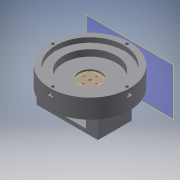
# Autodesk Inventor part: rotacion1_bottom
Saved by Autodesk Inventor 2018 (Build 220112000, 112)
## iProperties
Created: 2016-09-29
Part Number: rotacion1_bottom
Material: Generic
Document SubType Name: Modeling
Designer: Bardo91
Density: 1 g/cm^3
Appearance: Default
Author: Bardo91
Autodesk Inventor part; units mm, degrees
ref_plane "YZ Plane" through (0, 0, 0) normal (1, 0, 0) x (0, 1, 0)
ref_plane "XZ Plane" through (0, 0, 0) normal (0, 1, 0) x (-1, 0, 0)
ref_plane "XY Plane" through (0, 0, 0) normal (0, 0, 1) x (1, 0, 0)
sketch "Sketch1" plane through (0, 0, 0) normal (0, 0, 1) x (1, 0, 0)
  circle A0 centre (0, 0) radius 43
  circle A1 centre (0, 0) radius 50
  dimension "d0" = 86
  dimension "d1" = 100
  constraints: 2 centre point, 2 coincident
  measures "d0" diameter of A0
  measures "d1" diameter of A1
extrude "Extrusion1" add sketch "Sketch1" along normal blind 14
sketch "Sketch2" plane through (0, 0, 0) normal (0, 0, -1) x (-1, 0, 0)
  circle A0 centre (0, 0) radius 50.0172
  constraints: 1 centre point, 1 coincident
extrude "Extrusion2" add sketch "Sketch2" along normal blind 10
sketch "Sketch3" plane through (0, 0, -10) normal (0, 0, -1) x (-1, 0, 0)
  line L0 (0, 0) -> (0, 20)
  line L1 (0, 20) -> (-10, 20)
  line L2 (-10, 20) -> (-10, -20)
  line L3 (-10, -20) -> (31, -20)
  line L4 (31, -20) -> (31, 20)
  line L5 (31, 20) -> (0, 20)
  line L6 (-10, 20) -> (-10, 12.5)
  line L7 (-10, 12.5) -> (-17.5, 12.5)
  line L8 (-10, 12.5) -> (-10, 17.5)
  line L9 (-17.5, 17.5) -> (-17.5, 12.5)
  line L10 (-17.5, 12.5) -> (-17.5, -22.5)
  line L11 (-17.5, -22.5) -> (-32.5, -22.5)
  line L12 (-32.5, -22.5) -> (-32.5, 20)
  line L13 (-32.5, 20) -> (-17.5, 20)
  line L14 (31, -20) -> (31, -22.5)
  line L15 (31, -22.5) -> (38.5, -22.5)
  line L16 (38.5, -22.5) -> (38.5, 12.5)
  line L17 (38.5, 20) -> (31, 20)
  line L18 (-17.5, 20) -> (-10, 20)
  arc A0 (44.6514, -22.5) -> (45.8258, 20) centre (0, 0) ccw
  line L19 (38.5, -22.5) -> (44.6514, -22.5)
  line L20 (38.5, 20) -> (45.8258, 20)
  line L21 (31, 12.5) -> (38.5, 12.5)
  dimension "d6" = 20
  dimension "d7" = 10
  dimension "d8" = 40
  dimension "d9" = 41
  dimension "d10" = 7.5
  dimension "d11" = 7.5
  dimension "d13" = 35
  dimension "d14" = 15
  dimension "d16" = 7.5
  dimension "d24" = 2.5
  constraints: 44 end point, 10 perpendicular, 6 point on line, 5 vertical, 2 horizontal, 2 point on circle, 1 centre point, 1 coincident, 1 collinear
  measures "d6" distance of L0.start L0.end
  measures "d7" distance of L0.end L1.end
  measures "d8" distance of L1.end L2.end
  measures "d9" distance of L2.end L3.end
  measures "d10" distance of L1.end L6.end
  measures "d11" distance of L6.end L7.end
  measures "d13" distance of L7.end L10.end
  measures "d14" distance of L10.end L11.end
  measures "d16" distance of L14.end L15.end
  measures "d24" distance of L3.end L14.end
extrude "Extrusion3" add sketch "Sketch3" along normal blind 5 contours L5 L4 L3 L2 L1
extrude "Extrusion4" add sketch "Sketch3" along normal blind 25 contours L2 L7 L10 L11 L12 L13 L18 | L17 L20 A0 L19 L16 L21 L4
sketch "Sketch4" plane through (0, 0, -35) normal (0, 0, -1) x (-1, 0, 0)
  arc A0 (44.6514, -22.5) -> (45.8258, 20) centre (0, 0) ccw
  line L0 (45.8258, 20) -> (-32.5, 20)
  line L1 (-32.5, 20) -> (45.8258, 20) projected
  line L2 (-32.5, 20) -> (-32.5, -22.5)
  line L3 (-17.5, -22.5) -> (-32.5, -22.5) projected
  line L4 (-32.5, -22.5) -> (44.6514, -22.5)
  line L5 (38.5, -22.5) -> (44.6514, -22.5) projected
  dimension "d21" = 100
  constraints: 8 end point, 2 collinear, 2 point on circle, 1 centre point, 1 perpendicular
  measures "d21" diameter of A0
extrude "Extrusion5" add sketch "Sketch4" along normal blind 5
sketch "Sketch5" plane through (10, 12.5, -10) normal (0, -1, 0) x (1, 0, 0)
  line L0 (0, -25) -> (0, -5)
  line L1 (0, -5) -> (-41, -5)
  line L2 (0, -5) -> (-41, -5) projected
  line L3 (-20.5, -5) -> (-20.5, -25)
  line L4 (0, -5) -> (0, -25) projected
  line L5 (0, -15) -> (3, -15)
  line L6 (3, -15) -> (3, -20)
  line L7 (3, -15) -> (3, -10)
  circle A0 centre (3, -20) radius 3
  circle A1 centre (3, -10) radius 3
  line L8 (-41, -25) -> (-41, -5)
  line L9 (-41, -5) -> (0, -5)
  line L10 (-41, -5) -> (0, -5)
  line L11 (-41, -5) -> (-41, -25)
  line L12 (-41, -15) -> (-44, -15)
  line L13 (-44, -15) -> (-44, -20)
  line L14 (-44, -15) -> (-44, -10)
  circle A2 centre (-44, -20) radius 3
  circle A3 centre (-44, -10) radius 3
  point P0 (-10, 10)
  dimension "d25" = 3
  dimension "d26" = 5
  dimension "d27" = 5
  dimension "d28" = 6
  dimension "d29" = 6
  constraints: 26 end point, 9 symmetric about line, 4 centre point, 4 coincident, 4 vertical, 2 midpoint, 1 horizontal, 1 perpendicular, 2 other
  measures "d25" distance of L5.start L5.end
  measures "d26" distance of L5.end L6.end
  measures "d27" distance of L5.end L7.end
  measures "d28" diameter of A0
  measures "d29" diameter of A1
extrude "Extrusion6" cut sketch "Sketch5" against normal through all contours A0 | A1 | A2 | A3
sketch "Sketch6" plane through (0, 0, 14) normal (0, 0, 1) x (1, 0, 0)
  circle A0 centre (0, 0) radius 43 projected
  line L0 (0, 43) -> (0, 50.0172)
  circle A1 centre (0, 0) radius 50.0172 projected
  circle A2 centre (0, 46.5086) radius 1.75
  circle A3 centre (-46.5086, 0) radius 1.75
  circle A4 centre (0, -46.5086) radius 1.75
  circle A5 centre (46.5086, 0) radius 1.75
  dimension "d32" = 3.5
  dimension "d35" = 360
  constraints: 4 centre point, 2 end point, 2 vertical alignment, 1 midpoint, 11 other
  measures "d32" diameter of A2
extrude "Extrusion7" cut sketch "Sketch6" against normal through all contours A2 L0 | L0 A2 | A3 | A4 | A5
ref_plane "Work Plane1" through (0, 50.0172, 14) normal (0, 1, 0) x (-1, 0, 0)
sketch "Sketch12" plane through (0, 50.0172, 14) normal (0, 1, 0) x (-1, 0, 0)
  line L0 (0, 0) -> (0, -5)
  line L1 (0, -5) -> (3, -5)
  line L2 (3, -5) -> (3, -9)
  line L3 (3, -9) -> (-3, -9)
  line L4 (-3, -9) -> (-3, -5)
  line L5 (-3, -5) -> (0, -5)
  point P0 (0, -14)
  dimension "d51" = 5
  dimension "d52" = 3
  dimension "d53" = 4
  dimension "d54" = 6
  constraints: 12 end point, 5 perpendicular, 1 point on line, 1 vertical
  measures "d51" distance of L0.start L0.end
  measures "d52" distance of L0.end L1.end
  measures "d53" distance of L1.end L2.end
  measures "d54" distance of L2.end L3.end
extrude "Extrusion12" cut sketch "Sketch12" against normal blind 13
pattern_circular "Circular Pattern1" count 4 over 360 about axis through (0, 0, 0) along (0, 0, 1) of "Extrusion12"
sketch "Sketch14" plane through (0, 0, 0) normal (0, 0, 1) x (1, 0, 0)
  circle A0 centre (0, 0) radius 43
  circle A1 centre (0, 0) radius 33
  point P0 (10, 0)
  constraints: 2 centre point, 2 coincident
extrude "Extrusion14" add sketch "Sketch14" along normal blind 8
sketch "Sketch17" plane through (0, 0, -40) normal (0, 0, -1) x (-1, 0, 0)
  circle A0 centre (0, 0) radius 13
  dimension "d74" = 26
  constraints: 1 centre point, 1 coincident
  measures "d74" diameter of A0
extrude "Extrusion15" cut sketch "Sketch17" against normal blind 34
sketch "Sketch20" plane through (0, 0, 0) normal (0, 0, 1) x (1, 0, 0)
  circle A0 centre (0, 0) radius 13.5
  dimension "d103" = 27
  constraints: 1 centre point
  measures "d103" diameter of A0
ref_plane "Plano de trabajo2" through (0, 0, -2) normal (0, 0, 1) x (1, 0, 0)
sketch "Boceto21" plane through (0, 0, -2) normal (0, 0, 1) x (1, 0, 0)
  circle A0 centre (0, 8) radius 1
  circle A1 centre (8, 0) radius 1
  circle A2 centre (-8, 0) radius 1
  circle A3 centre (0, -8) radius 1
  circle A4 centre (0, 0) radius 1.5
  dimension "d96" = 2
  dimension "d97" = 2
  dimension "d98" = 2
  dimension "d99" = 2
  dimension "d100" = 3
  constraints: 5 centre point, 1 coincident
  measures "d96" diameter of A0
  measures "d97" diameter of A1
  measures "d98" diameter of A2
  measures "d99" diameter of A3
  measures "d100" diameter of A4
extrude "Extrusión19" cut sketch "Boceto21" against normal blind 8
extrude "Extrusión20" cut sketch "Sketch20" against normal blind 2
body "Solid1"
